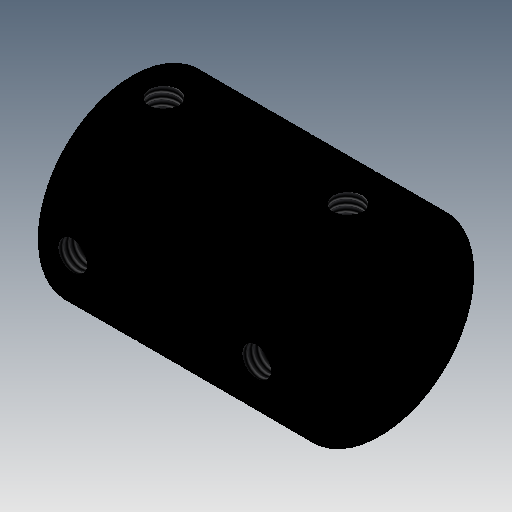
# Autodesk Inventor part: MCJN16-6-6_body
Saved by Autodesk Inventor 2019.4 (Build 234330000, 330)
## iProperties
Category: PARTsolutions
Company: MISUMI
Created: 2019-06-16
Part Number: MCJN16-6-6_body
Material: 一般
Catalog Web Link: www.cadenas.de
Description: MCJN_body-Couplings - Resin Type
Vendor: MISUMI
Document SubType Name: Modeling
Designer: psadmin
Manufacturer: MISUMI
Mass: 2.72436 g
Surface Area: 33.8371 cm^2
Volume: 2.72436 cm^3
Density: 1 g/cm^3
Appearance: PSOLRGB-0-0-0
PSOL_IDENT_0: {$CADENAS_DATA\23d-libs\misumi\metric\50_couplings\mcjn.prj},175 {VTYP=3D},{NB=MCJN16-6-6_body},{LIN
PSOL_IDENT_1: A=MCJN16-6-6},{NN=MCJN_body},{DATE=30.03.2018 07:24:16},{GEOMDATE=10.09.2008 06:56:00},{VERSION=},{L
PSOL_IDENT_2: INEID=40},{WBVAR=DD1,DD2},{WBNUMERIC=}  {NB=MCJN16-6-6_body},{LINA=MCJN16-6-6},{KT=DUMMY},{PN=MCJN16
PSOL_IDENT_3: -6-6},{MAT=Glass Fiber Reinforced PBT Resin},{AC=Set Screw},{TYPE=MCJN},{NO=16},{DD1=6},{DD1ALG1='6'
PSOL_IDENT_4: ,'6'},{DD1ALG2=6},{DD2=6},{DD2ALG1='3','3','3.2','3.2','4','4','5','5','6','6'},{DD2ALG2=6},{D=16},{
PSOL_IDENT_5: DIA=16.000},{L=21},{L1=21},{LL1=21},{LL11=21.000},{LL=5.5},{F=2.7},{M=M3X5},{T=0.25},{DL=6},{DR=6},{
PSOL_IDENT_6: TSIMD=3.000},{TSIMIN=2.459},{DIA1=2.8400},{L11=0.950},{L2=3.780},{L3=1.900},{TSS=3.000},{LSS=5.000}
NN: MCJN_body
NT: Couplings - Resin Type
NB: MCJN16-6-6_body
NBSYN: $TYPE.$NO.-$DD1.-$DD2._body
LINA: MCJN16-6-6
PN: MCJN16-6-6
MAT: Glass Fiber Reinforced PBT Resin
AC: Set Screw
NO: 16
DD1: 6
DD2: 6
D: 16
L: 21
LL: 5.5
F: 2.7
M: M3X5
T: 0.25
SUPPLIER: MISUMI
ARTICLENO: MCJN16-6-6_body
BOMINFO: MCJN16-6-6
CREATOR: CADENAS GmbH
Title: MCJN16-6-6
Author: Cadenas PARTsolutions
Comments: Couplings - Resin Type
Autodesk Inventor part; units mm, degrees
sketch "Sketch_1" plane through (0, 0, 0) normal (0, 0, 1) x (1, 0, 0)
  line L0 (21, 0) -> (0, 0)
  line L1 (0, 0) -> (0, 8)
  line L2 (0, 8) -> (21, 8)
  line L3 (21, 8) -> (21, 0)
  line L4 (21, 0) -> (0, 0)
  constraints: 10 end point
revolve "Revolution1" add sketch "Sketch_1" angle 360 about axis through (21, 0, 0) along (1, 0, 0)
sketch "Sketch_2" plane through (0, 0, 0) normal (0, 0, 1) x (1, 0, 0)
  line L0 (15.5, 0) -> (0, 0)
  line L1 (0, 0) -> (0, 3)
  line L2 (0, 3) -> (15.5, 3)
  line L3 (15.5, 3) -> (15.5, 0)
  line L4 (15.5, 0) -> (0, 0)
  constraints: 10 end point
revolve "Revolution2" cut sketch "Sketch_2" angle 360 about axis through (15.5, 0, 0) along (1, 0, 0)
sketch "Sketch3" plane through (21, 0, 0) normal (1, 0, 0) x (0, 0, -1)
  point P0 (0, 0)
hole "Hole1" at (21, 0, 0) direction (-1, 0, 0) diameter 6 depth 5.5
sketch "Sketch_4" plane through (0, 0, 0) normal (0, 0, 1) x (1, 0, 0)
  arc A0 (5.5, 1.9) -> (6.45, 1.9) centre (5.975, 1.9) ccw
  line L0 (6.45, 1.9) -> (6.45, 8)
  line L1 (6.45, 8) -> (9.125, 8)
  line L2 (9.125, 8) -> (9.125, 1.9)
  arc A1 (9.125, 1.9) -> (10.075, 1.9) centre (9.6, 1.9) ccw
  line L3 (10.075, 1.9) -> (10.075, 8)
  line L4 (10.075, 8) -> (12.65, 8)
  line L5 (12.65, 8) -> (12.65, 1.9)
  arc A2 (12.65, 1.9) -> (13.6, 1.9) centre (13.125, 1.9) ccw
  line L6 (13.6, 1.9) -> (13.6, 9.6)
  line L7 (13.6, 9.6) -> (5.5, 9.6)
  line L8 (5.5, 9.6) -> (5.5, 1.9)
  constraints: 18 end point, 6 point on circle, 3 centre point
extrude "Extrusion1" cut sketch "Sketch_4" along normal mid plane 16
sketch "Sketch_5" plane through (0, 0, 0) normal (0, 0, 1) x (1, 0, 0)
  line L0 (5.5, -1.9) -> (5.5, -9.6)
  line L1 (5.5, -9.6) -> (13.6, -9.6)
  line L2 (13.6, -9.6) -> (13.6, -1.9)
  arc A0 (13.6, -1.9) -> (12.65, -1.9) centre (13.125, -1.9) ccw
  line L3 (12.65, -1.9) -> (12.65, -8)
  line L4 (12.65, -8) -> (10.075, -8)
  line L5 (10.075, -8) -> (10.075, -1.9)
  arc A1 (10.075, -1.9) -> (9.125, -1.9) centre (9.6, -1.9) ccw
  line L6 (9.125, -1.9) -> (9.125, -8)
  line L7 (9.125, -8) -> (6.45, -8)
  line L8 (6.45, -8) -> (6.45, -1.9)
  arc A2 (6.45, -1.9) -> (5.5, -1.9) centre (5.975, -1.9) ccw
  constraints: 18 end point, 6 point on circle, 3 centre point
extrude "Extrusion2" cut sketch "Sketch_5" along normal mid plane 16
sketch "Sketch_6" plane through (0, 0, 0) normal (0, 1, 0) x (-1, 0, 0)
  arc A0 (-7.4, -1.9) -> (-8.35, -1.9) centre (-7.875, -1.9) ccw
  line L0 (-8.35, -1.9) -> (-8.35, -8)
  line L1 (-8.35, -8) -> (-11.025, -8)
  line L2 (-11.025, -8) -> (-11.025, -1.9)
  arc A1 (-11.025, -1.9) -> (-11.975, -1.9) centre (-11.5, -1.9) ccw
  line L3 (-11.975, -1.9) -> (-11.975, -8)
  line L4 (-11.975, -8) -> (-14.55, -8)
  line L5 (-14.55, -8) -> (-14.55, -1.9)
  arc A2 (-14.55, -1.9) -> (-15.5, -1.9) centre (-15.025, -1.9) ccw
  line L6 (-15.5, -1.9) -> (-15.5, -9.6)
  line L7 (-15.5, -9.6) -> (-7.4, -9.6)
  line L8 (-7.4, -9.6) -> (-7.4, -1.9)
  constraints: 18 end point, 6 point on circle, 3 centre point
extrude "Extrusion3" cut sketch "Sketch_6" along normal mid plane 16
sketch "Sketch_7" plane through (0, 0, 0) normal (0, 1, 0) x (-1, 0, 0)
  line L0 (-7.4, 1.9) -> (-7.4, 9.6)
  line L1 (-7.4, 9.6) -> (-15.5, 9.6)
  line L2 (-15.5, 9.6) -> (-15.5, 1.9)
  arc A0 (-15.5, 1.9) -> (-14.55, 1.9) centre (-15.025, 1.9) ccw
  line L3 (-14.55, 1.9) -> (-14.55, 8)
  line L4 (-14.55, 8) -> (-11.975, 8)
  line L5 (-11.975, 8) -> (-11.975, 1.9)
  arc A1 (-11.975, 1.9) -> (-11.025, 1.9) centre (-11.5, 1.9) ccw
  line L6 (-11.025, 1.9) -> (-11.025, 8)
  line L7 (-11.025, 8) -> (-8.35, 8)
  line L8 (-8.35, 8) -> (-8.35, 1.9)
  arc A2 (-8.35, 1.9) -> (-7.4, 1.9) centre (-7.875, 1.9) ccw
  constraints: 18 end point, 6 point on circle, 3 centre point
extrude "Extrusion4" cut sketch "Sketch_7" along normal mid plane 16
sketch "Sketch_8" plane through (2.7, 0, 0) normal (1, 0, 0) x (0, 0, -1)
  line L0 (0, 0) -> (0, 8)
  line L1 (0, 8) -> (1.5, 8)
  line L2 (1.5, 8) -> (1.2295, 7.7295)
  line L3 (1.2295, 7.7295) -> (1.2295, 0)
  line L4 (1.2295, 0) -> (0, 0)
  line L5 (0, 0) -> (0, 8)
  constraints: 12 end point
revolve "Revolution3" cut sketch "Sketch_8" angle 360 about axis through (2.7, 0, 0) along (0, -1, 0)
thread "Thread1" size "M3x0.5" class "6H" standard "ISO Metric profile" length 4.7295
sketch "Sketch_9" plane through (2.7, 0, 0) normal (1, 0, 0) x (0, 0, -1)
  line L0 (0, 0) -> (-8, 0)
  line L1 (-8, 0) -> (-8, 1.5)
  line L2 (-8, 1.5) -> (-7.7295, 1.2295)
  line L3 (-7.7295, 1.2295) -> (0, 1.2295)
  line L4 (0, 1.2295) -> (0, 0)
  line L5 (0, 0) -> (-8, 0)
  constraints: 12 end point
revolve "Revolution4" cut sketch "Sketch_9" angle 360 about axis through (2.7, 0, 0) along (0, 0, -1)
thread "Thread2" size "M3x0.5" class "6H" standard "ISO Metric profile" length 4.7295
sketch "Sketch_10" plane through (18.3, 0, 0) normal (1, 0, 0) x (0, 0, -1)
  line L0 (0, 0) -> (0, 8)
  line L1 (0, 8) -> (1.5, 8)
  line L2 (1.5, 8) -> (1.2295, 7.7295)
  line L3 (1.2295, 7.7295) -> (1.2295, 0)
  line L4 (1.2295, 0) -> (0, 0)
  line L5 (0, 0) -> (0, 8)
  constraints: 12 end point
revolve "Revolution5" cut sketch "Sketch_10" angle 360 about axis through (18.3, 0, 0) along (0, -1, 0)
thread "Thread3" size "M3x0.5" class "6H" standard "ISO Metric profile" length 4.7295
sketch "Sketch_11" plane through (18.3, 0, 0) normal (1, 0, 0) x (0, 0, -1)
  line L0 (0, 0) -> (-8, 0)
  line L1 (-8, 0) -> (-8, 1.5)
  line L2 (-8, 1.5) -> (-7.7295, 1.2295)
  line L3 (-7.7295, 1.2295) -> (0, 1.2295)
  line L4 (0, 1.2295) -> (0, 0)
  line L5 (0, 0) -> (-8, 0)
  constraints: 12 end point
revolve "Revolution6" cut sketch "Sketch_11" angle 360 about axis through (18.3, 0, 0) along (0, 0, -1)
thread "Thread4" size "M3x0.5" class "6H" standard "ISO Metric profile" length 4.7295
ref_plane "cp1_XY" through (2.7, 8, 0) normal (0, 1, 0) x (1, 0, 0)
ref_plane "cp1_YZ" through (2.7, 8, 0) normal (1, 0, 0) x (0, 0, -1)
ref_plane "cp1_ZX" through (2.7, 8, 0) normal (0, 0, -1) x (0, 1, 0)
ref_plane "cp2_XY" through (18.3, 8, 0) normal (0, 1, 0) x (1, 0, 0)
ref_plane "cp2_YZ" through (18.3, 8, 0) normal (1, 0, 0) x (0, 0, -1)
ref_plane "cp2_ZX" through (18.3, 8, 0) normal (0, 0, -1) x (0, 1, 0)
ref_plane "cp3_XY" through (2.7, 0, 8) normal (0, 0, 1) x (1, 0, 0)
ref_plane "cp3_YZ" through (2.7, 0, 8) normal (1, 0, 0) x (0, 1, 0)
ref_plane "cp3_ZX" through (2.7, 0, 8) normal (0, 1, 0) x (0, 0, 1)
ref_plane "cp4_XY" through (18.3, 0, 8) normal (0, 0, 1) x (1, 0, 0)
ref_plane "cp4_YZ" through (18.3, 0, 8) normal (1, 0, 0) x (0, 1, 0)
ref_plane "cp4_ZX" through (18.3, 0, 8) normal (0, 1, 0) x (0, 0, 1)
body "Solid1"
